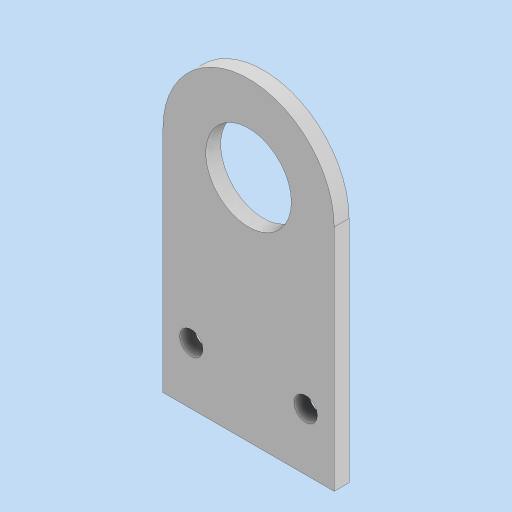
# Autodesk Inventor part: ArmPlateBase
Saved by Autodesk Inventor 2024 (Build 280153000, 153)
## iProperties
Created: 2024-01-11
Part Number: ArmPlateBase
Material: Generic
Document SubType Name: Modeling
Designer: megan
Density: 1 g/cm^3
Appearance: Default
Author: megan
Autodesk Inventor part; units mm, degrees
ref_plane "YZ Plane" through (0, 0, 0) normal (1, 0, 0) x (0, 1, 0)
ref_plane "XZ Plane" through (0, 0, 0) normal (0, 1, 0) x (-1, 0, 0)
ref_plane "XY Plane" through (0, 0, 0) normal (0, 0, 1) x (1, 0, 0)
sketch "Sketch1" plane through (0, 0, 0) normal (0, 0, 1) x (1, 0, 0)
  arc A0 (19, 0) -> (-19, 0) centre (0, 0) ccw
  circle A1 centre (0, 0) radius 9.5
  line L0 (-19, -50.8) -> (19, -50.8)
  line L1 (19, -50.8) -> (19, 0)
  line L2 (-19, 0) -> (-19, -50.8)
  line L3 (0, -64.76) -> (0, 32.96) projected
  circle A2 centre (-12.7, -38.1) radius 2.5781
  circle A3 centre (12.7, -38.1) radius 2.5781
  dimension "d0" = 38
  dimension "d1" = 19
  dimension "d10" = 5.1562
  dimension "d11" = 5.1562
  dimension "d12" = 12.7
  dimension "d13" = 12.7
  dimension "d14" = 12.7
  dimension "d15" = 12.7
  dimension "d16" = 50.8
  constraints: 6 end point, 4 centre point, 3 parallel, 2 coincident, 2 point on circle, 1 perpendicular, 1 tangent
  measures "d0" diameter of A0
  measures "d1" diameter of A1
  measures "d10" diameter of A2
  measures "d11" diameter of A3
  measures "d12" distance from line of L0 A2.centre
  measures "d13" distance from line of L0 A3.centre
  measures "d14" distance from line of L3 A2.centre
  measures "d15" distance from line of L3 A3.centre
  measures "d16" distance from line of L0 point (0, 0)
extrude "Extrusion1" add sketch "Sketch1" along normal blind 3.302 contours L1 L0 L3 A1 A0 | L3 A1 L0 L2 A0
equation "\"d0\" = 2 * d1"
body "Solid1"
